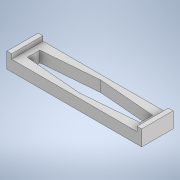
# Autodesk Inventor part: testing deadbolt arm adapter
Saved by Autodesk Inventor 2022 (Build 260153000, 153)
## iProperties
Created: 2021-11-09
Part Number: testing deadbolt arm adapter
Material: Generic
Document SubType Name: Modeling
Designer: a-dubs
Density: 1 g/cm^3
Appearance: Default
Author: a-dubs
Autodesk Inventor part; units mm, degrees
ref_plane "YZ Plane" through (0, 0, 0) normal (1, 0, 0) x (0, 1, 0)
ref_plane "XZ Plane" through (0, 0, 0) normal (0, 1, 0) x (-1, 0, 0)
ref_plane "XY Plane" through (0, 0, 0) normal (0, 0, 1) x (1, 0, 0)
sketch "Sketch1" plane through (0, 0, 0) normal (0, 1, 0) x (-1, 0, 0)
  line L0 (0, 0) -> (0, 38)
  line L1 (0, 38) -> (0, 43)
  line L2 (0, 38) -> (2, 38)
  line L3 (2, 38) -> (-2, 38)
  line L4 (-2, 38) -> (0, 43)
  line L5 (2, 38) -> (0, 43)
  line L6 (-2, 38) -> (-2, 2)
  line L7 (2, 2) -> (2, 38)
  line L8 (-2, 2) -> (-2, 3)
  line L9 (2, 2) -> (2, 0)
  line L10 (-2, 2) -> (-2, 0)
  line L11 (-2, 0) -> (2, 0)
  line L12 (0, 0) -> (-2, 1)
  line L13 (0, 38) -> (0, 42)
  line L14 (0, 42) -> (-0.4, 42)
  line L15 (0.4, 42) -> (0, 42)
  line L16 (0, 0) -> (0, 10)
  line L17 (0, 10) -> (0, 0)
  line L18 (0, 0) -> (-40, 0)
  line L19 (-40, 0) -> (-40, -10)
  line L20 (-40, 10) -> (40, 10)
  line L21 (40, 10) -> (40, -10)
  line L22 (40, -10) -> (-40, -10)
  line L23 (-40, -10) -> (-40, 10)
  line L24 (40, -10) -> (38, -10)
  line L25 (38, -10) -> (43, -10)
  line L26 (43, -10) -> (43, 10)
  line L27 (43, 10) -> (38, 10)
  line L28 (38, 10) -> (38, -10)
  line L29 (-40, -10) -> (-38, -10)
  line L30 (-38, -10) -> (-43, -10)
  line L31 (-43, -10) -> (-43, 10)
  line L32 (-43, 10) -> (-38, 10)
  line L33 (-38, 10) -> (-38, -10)
  point P0 (0, 2)
  dimension "d0" = 38
  dimension "d1" = 5
  dimension "d2" = 2
  dimension "d3" = 4
  dimension "d6" = 1
  dimension "d30" = 4
  dimension "d31" = 10
  dimension "d32" = 40
  dimension "d33" = 10
  dimension "d34" = 80
  dimension "d37" = 2
  dimension "d38" = 5
  dimension "d39" = 2
  dimension "d40" = 5
  constraints: 68 end point, 10 point on line, 8 equal length, 6 perpendicular, 5 horizontal, 4 vertical, 1 midpoint
  measures "d0" distance of L0.start L0.end
  measures "d1" distance of L0.end L1.end
  measures "d2" distance of L0.end L2.end
  measures "d3" distance of L2.end L3.end
  measures "d6" distance of L6.end L8.end
  measures "d30" distance of L0.end L13.end
  measures "d31" distance of L0.start L16.end
  measures "d32" distance of L0.start L18.end
  measures "d33" distance of L18.end L19.end
  measures "d34" distance of L21.end L22.end
  measures "d37" distance of L21.end L24.end
  measures "d38" distance of L27.end L26.end
  measures "d39" distance of L22.end L29.end
  measures "d40" distance of L31.end L32.end
extrude "Extrusion1" add sketch "Sketch1" along normal blind 7 contours L12 L10 L6 L20 L0 | L11 L9 L7 L20 L28 L22 L33 L18 | L0 L20 L7 L9 L11 | L11 L10 L12 | L18 L33 L20 L6 L10 | L33 L22 L19 L18 | L18 L23 L20 L33 | L20 L21 L22 L28 | L19 L30 L31 L32 L23 | L27 L26 L25 L21
sketch "Sketch4" plane through (0, 7, 0) normal (0, 1, 0) x (1, 0, 0)
  circle A0 centre (0, 0) radius 1.5
  line L0 (0, 0) -> (-36, 0)
  line L1 (-36, 0) -> (-36, -4)
  line L2 (0, 0) -> (0, -7)
  line L3 (-36, -4) -> (0, -7)
  line L4 (-36, 0) -> (-36, 4)
  line L5 (0, 0) -> (0, 7)
  line L6 (-36, 4) -> (0, 7)
  line L7 (0, 0) -> (36, 0)
  line L8 (36, 0) -> (36, -4)
  line L9 (36, -4) -> (0, -7)
  line L10 (36, 4) -> (0, 7)
  line L11 (36, 0) -> (36, 4)
  dimension "d20" = 3
  dimension "d26" = 36
  dimension "d28" = 4
  dimension "d29" = 7
  constraints: 24 end point, 5 symmetric about line, 2 vertical, 1 centre point, 1 coincident, 1 horizontal
  measures "d20" diameter of A0
  measures "d26" distance of L0.start L0.end
  measures "d28" distance of L0.end L1.end
  measures "d29" distance of L0.start L2.end
extrude "Extrusion5" cut sketch "Sketch4" against normal through all
extrude "Extrusion6" add sketch "Sketch1" along normal blind 3 from surface at 7 contours L19 L30 L31 L32 L23 | L27 L26 L25 L21
body "Solid1"
